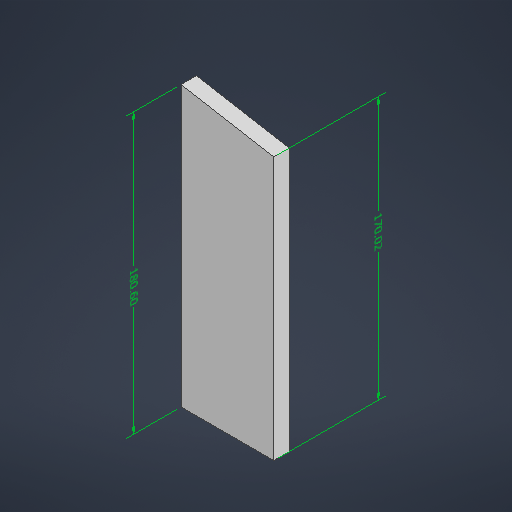
# Autodesk Inventor part: stand
Saved by Autodesk Inventor 2026.2 (Build 302298000, 298)
## iProperties
Created: 2026-02-23
Part Number: stand
Material: Generic
Document SubType Name: Sheet Metal
Designer: danda
Density: 1 g/cm^3
Sheet Metal Rule: Default_mm
Appearance: Default
Author: danda
Autodesk Inventor part; units mm, degrees
ref_plane "YZ Plane" through (0, 0, 0) normal (1, 0, 0) x (0, 1, 0)
ref_plane "XZ Plane" through (0, 0, 0) normal (0, 1, 0) x (-1, 0, 0)
ref_plane "XY Plane" through (0, 0, 0) normal (0, 0, 1) x (1, 0, 0)
sketch "Sketch1" plane through (0, 0, 0) normal (0, 0, 1) x (1, 0, 0)
  line L0 (19.2985, -19.7179) -> (19.2985, 160.8861)
  line L1 (19.2985, -19.7179) -> (79.2985, -19.7179)
  line L2 (79.2985, -19.7179) -> (79.2985, 150.3065)
  line L3 (79.2985, -19.7179) -> (19.2985, -19.7179)
  line L4 (79.2985, -19.7179) -> (19.2985, -19.7179)
  line L5 (19.2985, 160.8861) -> (79.2985, 150.3065)
  point P0 (0, 0)
  dimension "d3" = 60
  dimension "d23" = 80
  dimension "d24" = 180.604
  constraints: 12 end point, 2 vertical, 1 perpendicular
  measures "d3" distance of L0.start L1.end
  measures "d23" angle of L0 L5
  measures "d24" distance of L0.end L0.start
extrude "Extrusion1" add sketch "Sketch1" along normal mid plane 10
equation "\"BendRadius\" = Thickness"
equation "\"BendReliefWidth\" = Thickness"
equation "\"BendReliefDepth\" = 0.5 * Thickness"
equation "\"CornerReliefSize\" = 4 * Thickness"
equation "\"MinimumRemnant\" = 2 * Thickness"
equation "\"TransitionRadius\" = BendRadius"
equation "\"JacobiRadiusSize\" = BendRadius"
equation "\"GapSize\" = Thickness"
equation "\"Thickness\" = 0.5"
body "Solid1"
